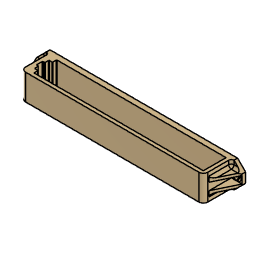
Porta Fusivel single v1 (Autodesk Fusion 360 design; units mm, degrees)
Autodesk Fusion 360 part; units mm, degrees
sketch "Sketch1" plane through (0, 0, 0) normal (0, 0, 1) x (1, 0, 0)
  line L0 (0, 0) -> (197, 0)
  line L1 (197, 0) -> (197, 25.5)
  line L2 (197, 25.5) -> (0, 25.5)
  line L3 (0, 25.5) -> (0, 0)
  line L4 (6.5, 25.5) -> (6.5, 20.8)
  line L5 (6.5, 20.8) -> (2.5, 20.8)
  line L6 (0, 12.75) -> (197, 12.75) construction
  line L7 (197, 17.5) -> (188, 17.5)
  line L8 (188, 17.5) -> (188, 8)
  line L9 (188, 8) -> (197, 8)
  line L10 (6.5, 4.7) -> (2.5, 4.7)
  line L11 (6.5, 0) -> (6.5, 4.7)
  line L12 (2.5, 20.8) -> (2.5, 16.25)
  line L13 (2.5, 16.25) -> (0, 16.25)
  line L14 (2.5, 4.7) -> (2.5, 9.25)
  line L15 (2.5, 9.25) -> (0, 9.25)
  line L16 (0, 25.5) -> (0, 51)
  line L17 (0, 51) -> (197, 51)
  line L18 (6.5, 46.3) -> (2.5, 46.3)
  line L19 (6.5, 51) -> (6.5, 46.3)
  line L20 (2.5, 41.75) -> (0, 41.75)
  line L21 (2.5, 46.3) -> (2.5, 41.75)
  line L22 (6.5, 25.5) -> (6.5, 30.2)
  line L23 (6.5, 30.2) -> (2.5, 30.2)
  line L24 (2.5, 30.2) -> (2.5, 34.75)
  line L25 (2.5, 34.75) -> (0, 34.75)
  line L26 (197, 33.5) -> (188, 33.5)
  line L27 (188, 33.5) -> (188, 43)
  line L28 (188, 43) -> (197, 43)
  line L29 (197, 51) -> (197, 25.5)
  line L30 (201, -4) -> (201, 25.5)
  line L31 (201, 55) -> (201, 25.5)
  line L32 (-4, 55) -> (201, 55)
  line L33 (-4, 25.5) -> (-4, 55)
  line L34 (-4, 25.5) -> (-4, -4)
  line L35 (-4, -4) -> (201, -4)
  line L36 (201, 21.5) -> (-4, 21.5)
  point P0 (0, 25.5)
  dimension "d1" = 25.5
  dimension "d2" = 197
  dimension "d5" = 4.7
  dimension "d6" = 4
  dimension "d7" = 9
  dimension "d8" = 9.5
  dimension "d9" = 2.5
  dimension "d10" = 7
  dimension "d19" = 4
  dimension "d74" = 4
  constraint horizontal L0
  constraint vertical L1
  constraint horizontal L2
  constraint vertical L3
  constraint coincident L0.start L3.end
  constraint coincident P0 L2
  constraint coincident P0 L3
  constraint coincident L3.end L0
  constraint coincident L0.start L3
  constraint coincident L2 L4.start
  constraint perpendicular L2 L4
  constraint perpendicular L3 L5
  constraint midpoint L3 L6.start
  constraint perpendicular L3 L6
  constraint midpoint L1 L6.end
  constraint coincident L1 L7.start
  constraint perpendicular L1 L7
  constraint perpendicular L6 L8
  constraint coincident L1 L9.end
  constraint perpendicular L1 L9
  constraint symmetric L6 L7 L9
  constraint symmetric L4.start L6 L11.start
  constraint symmetric L4.end L6 L10.start
  constraint symmetric L5.end L6 L10.end
  constraint perpendicular L5 L12
  constraint coincident L3 L13.end
  constraint perpendicular L3 L13
  constraint symmetric L6 L12.end L14.end
  constraint symmetric L6 L13.end L15.end
  constraint coincident P0 L2.end
  constraint coincident L0.end L1.start
  constraint symmetric L2 P0 L3.start
  constraint symmetric L2 L1.end L29.end
  constraint symmetric L2 L0.end L17.end
  constraint symmetric L2 L0.start L16.end
  constraint symmetric L2 L4.start L22.start
  constraint symmetric L2 L4.end L22.end
  constraint symmetric L2 L5.end L23.end
  constraint symmetric L2 L7.start L26.start
  constraint symmetric L2 L7.end L26.end
  constraint symmetric L2 L8.end L27.end
  constraint symmetric L2 L9.end L28.end
  constraint symmetric L2 L10.start L18.start
  constraint symmetric L2 L10.end L18.end
  constraint symmetric L2 L11.start L19.start
  constraint symmetric L2 L12.end L24.end
  constraint symmetric L2 L13.end L25.end
  constraint symmetric L2 L14.end L20.start
  constraint symmetric L2 L15.end L20.end
  constraint coincident L31 L36.start
  constraint coincident L33 L36.end
  constraint perpendicular L33 L36
  measures "d1" distance of L0.start P0
  measures "d2" distance of L1 L3
  measures "d5" distance of L4.start L4.end
  measures "d6" distance of L4.end L5.end
  measures "d7" distance of L7.start L7.end
  measures "d8" distance of L7.end L8.end
  measures "d9" distance of L12.end L13.end
  measures "d10" distance of L13 L15
  measures "d74" distance of L2 L36
extrude "Extrude1" add sketch "Sketch1" against normal blind 2 contours L1 L3 L16 L17 L29 L30 L31 L32 L33 L34 L36 | L2 L3 L4 L36 | L2 L16 L22 L23 L24 L25 | L1 L2 L4 L36 | L16 L17 L18 L19 L20 L21 | L26 L27 L28 L29
extrude "Extrude2" add sketch "Sketch1" along normal blind 9 contours L26 L27 L28 L29
extrude "Extrude3" add sketch "Sketch1" along normal blind 27 contours L1 L3 L16 L17 L29 L30 L31 L32 L33 L34 L36 | L2 L3 L4 L36 | L2 L16 L22 L23 L24 L25 | L1 L2 L4 L36 | L16 L17 L18 L19 L20 L21
fillet "Fillet1" radius 0.5 16 edges at (2.5, 34.75, 12.5) (2.5, 30.2, 12.5) (6.5, 46.3, 12.5) (2.5, 46.3, 12.5) (2.5, 41.75, 12.5) (6.5, 51, 12.5) (0, 41.75, 12.5) (0, 34.75, 12.5) (188, 43, 3.5) (188, 33.5, 3.5) (197, 51, 12.5) (197, 25.5, 12.5) (197, 43, 3.5) (197, 33.5, 3.5) (6.5, 25.5, 12.5) (6.5, 30.2, 12.5)
fillet "Fillet3" radius 5 2 edges at (201, 21.5, 12.5) (-4, 21.5, 12.5)
sketch "Sketch3" plane through (0, 0, -2) normal (0, 0, -1) x (1, 0, 0)
  line L0 (-4, -26.5) -> (-4, -55)
  line L1 (-4, -55) -> (201, -55)
  line L2 (201, -55) -> (201, -26.5)
  line L3 (197, -43.5) -> (197, -50.5)
  line L4 (196.5, -33.5) -> (188.5, -33.5)
  arc A0 (188.5, -33.5) -> (188, -34) centre (188.5, -34) ccw
  line L5 (188, -34) -> (188, -42.5)
  arc A1 (188, -42.5) -> (188.5, -43) centre (188.5, -42.5) ccw
  line L6 (188.5, -43) -> (196.5, -43)
  line L7 (196.5, -51) -> (7, -51)
  arc A2 (6.5, -50.5) -> (7, -51) centre (7, -50.5) ccw
  line L8 (6.5, -50.5) -> (6.5, -46.8)
  arc A3 (6.5, -46.8) -> (6, -46.3) centre (6, -46.8) ccw
  line L9 (6, -46.3) -> (3, -46.3)
  arc A4 (2.5, -45.8) -> (3, -46.3) centre (3, -45.8) ccw
  line L10 (2.5, -45.8) -> (2.5, -42.25)
  arc A5 (2.5, -42.25) -> (2, -41.75) centre (2, -42.25) ccw
  line L11 (2, -41.75) -> (0.5, -41.75)
  arc A6 (0, -41.25) -> (0.5, -41.75) centre (0.5, -41.25) ccw
  line L12 (0, -41.25) -> (0, -35.25)
  arc A7 (0.5, -34.75) -> (0, -35.25) centre (0.5, -35.25) ccw
  line L13 (0.5, -34.75) -> (2, -34.75)
  arc A8 (2, -34.75) -> (2.5, -34.25) centre (2, -34.25) ccw
  line L14 (2.5, -34.25) -> (2.5, -30.7)
  arc A9 (3, -30.2) -> (2.5, -30.7) centre (3, -30.7) ccw
  line L15 (3, -30.2) -> (6, -30.2)
  line L16 (6.5, -29.7) -> (6.5, -26)
  line L17 (7, -25.5) -> (196.5, -25.5)
  line L18 (196, -21.5) -> (1, -21.5)
  arc A10 (196.5, -51) -> (197, -50.5) centre (196.5, -50.5) ccw
  arc A11 (197, -26) -> (196.5, -25.5) centre (196.5, -26) ccw
  line L19 (197, -26) -> (197, -33)
  arc A12 (1, -21.5) -> (-4, -26.5) centre (1, -26.5) ccw
  arc A13 (201, -26.5) -> (196, -21.5) centre (196, -26.5) ccw
  arc A14 (6, -30.2) -> (6.5, -29.7) centre (6, -29.7) ccw
  arc A15 (7, -25.5) -> (6.5, -26) centre (7, -26) ccw
  arc A16 (196.5, -33.5) -> (197, -33) centre (196.5, -33) ccw
  arc A17 (197, -43.5) -> (196.5, -43) centre (196.5, -43.5) ccw
  line L20 (188.5, -44.65) -> (195.35, -44.65)
  line L21 (195.35, -44.65) -> (195.35, -49.35)
  line L22 (195.35, -49.35) -> (8.15, -49.35)
  line L23 (8.15, -49.35) -> (8.15, -46.8)
  arc A18 (8.15, -46.8) -> (6, -44.65) centre (6, -46.8) ccw
  line L24 (6, -44.65) -> (4.15, -44.65)
  line L25 (4.15, -44.65) -> (4.15, -42.25)
  arc A19 (4.15, -42.25) -> (2, -40.1) centre (2, -42.25) ccw
  line L26 (2, -40.1) -> (1.65, -40.1)
  line L27 (1.65, -40.1) -> (1.65, -36.4)
  line L28 (1.65, -36.4) -> (2, -36.4)
  arc A20 (2, -36.4) -> (4.15, -34.25) centre (2, -34.25) ccw
  line L29 (4.15, -34.25) -> (4.15, -31.85)
  line L30 (4.15, -31.85) -> (6, -31.85)
  arc A21 (6, -31.85) -> (8.15, -29.7) centre (6, -29.7) ccw
  line L31 (8.15, -29.7) -> (8.15, -27.15)
  line L32 (8.15, -27.15) -> (195.35, -27.15)
  line L33 (195.35, -27.15) -> (195.35, -31.85)
  line L34 (195.35, -31.85) -> (188.5, -31.85)
  arc A22 (188.5, -31.85) -> (186.35, -34) centre (188.5, -34) ccw
  line L35 (186.35, -34) -> (186.35, -42.5)
  arc A23 (186.35, -42.5) -> (188.5, -44.65) centre (188.5, -42.5) ccw
  dimension "d24" = 2
  dimension "d77" = 1.65
extrude "Extrude4" add sketch "Sketch3" against normal blind 2 contours L3 L4 A0 L5 A1 L6 L7 A2 L8 A3 L9 A4 L10 A5 L11 A6 L12 A7 L13 A8 L14 A9 L15 L16 L17 A10 A11 L19 A14 A15 A16 A17
sketch "Sketch4" plane through (0, 0, 27) normal (0, 0, 1) x (-1, 0, 0)
  arc A0 (-2, -41.75) -> (-2.5, -42.25) centre (-2, -42.25) ccw
  line L0 (-2.5, -42.25) -> (-2.5, -45.8)
  arc A1 (-3, -46.3) -> (-2.5, -45.8) centre (-3, -45.8) ccw
  line L1 (-3, -46.3) -> (-6, -46.3)
  arc A2 (-6, -46.3) -> (-6.5, -46.8) centre (-6, -46.8) ccw
  line L2 (-6.5, -46.8) -> (-6.5, -50.5)
  arc A3 (-7, -51) -> (-6.5, -50.5) centre (-7, -50.5) ccw
  line L3 (-7, -51) -> (-196.5, -51)
  line L4 (-197, -50.5) -> (-197, -26)
  line L5 (-6.5, -26) -> (-6.5, -29.7)
  line L6 (-6, -30.2) -> (-3, -30.2)
  arc A4 (-2.5, -30.7) -> (-3, -30.2) centre (-3, -30.7) ccw
  line L7 (-2.5, -30.7) -> (-2.5, -34.25)
  arc A5 (-2.5, -34.25) -> (-2, -34.75) centre (-2, -34.25) ccw
  line L8 (-2, -34.75) -> (-0.5, -34.75)
  arc A6 (0, -35.25) -> (-0.5, -34.75) centre (-0.5, -35.25) ccw
  line L9 (0, -35.25) -> (0, -41.25)
  arc A7 (-0.5, -41.75) -> (0, -41.25) centre (-0.5, -41.25) ccw
  line L10 (-0.5, -41.75) -> (-2, -41.75)
  line L11 (-201, -26.5) -> (-201, -55)
  line L12 (-201, -55) -> (4, -55)
  line L13 (4, -55) -> (4, -26.5)
  line L14 (-7, -51) -> (4, -51)
  line L15 (-196.5, -51) -> (-201, -51)
  line L16 (-1, -21.5) -> (-196, -21.5)
  line L17 (-196.5, -25.5) -> (-7, -25.5)
  arc A8 (-197, -50.5) -> (-196.5, -51) centre (-196.5, -50.5) ccw
  arc A9 (-196.5, -25.5) -> (-197, -26) centre (-196.5, -26) ccw
  arc A10 (4, -26.5) -> (-1, -21.5) centre (-1, -26.5) ccw
  arc A11 (-196, -21.5) -> (-201, -26.5) centre (-196, -26.5) ccw
  arc A12 (-6.5, -29.7) -> (-6, -30.2) centre (-6, -29.7) ccw
  arc A13 (-6.5, -26) -> (-7, -25.5) centre (-7, -26) ccw
  constraint coincident A3.start L3.start
  constraint coincident L13 L14.end
  constraint tangent A3 L14
  constraint coincident L3.end L15.start
  constraint coincident L11 L15.end
extrude "Extrude8" add 1 faces at (132.6667, 55, 17.3333) along direction (0, 1, 0) blind 2
sketch "Sketch6" plane through (0, 57, 0) normal (0, 1, 0) x (-1, 0, 0)
  line L0 (-201, 27) -> (-201, -2)
  line L1 (-201, -2) -> (4, -2)
  line L2 (4, -2) -> (4, 27)
  line L3 (4, 27) -> (-201, 27)
  line L4 (4, 27) -> (7, 27)
  line L5 (7, 27) -> (16, 18)
  line L6 (16, 18) -> (16, 14.25)
  line L7 (16, 14.25) -> (10, 14.25)
  arc A0 (10, 14.25) -> (10, 10.75) centre (10, 12.5) ccw
  line L8 (10, 12.5) -> (4, 12.5) construction
  line L9 (4, -2) -> (7, -2)
  line L10 (7, -2) -> (16, 7)
  line L11 (16, 7) -> (16, 10.75)
  line L12 (16, 10.75) -> (10, 10.75)
  line L13 (-98.5, 27) -> (-98.5, 53.5133) construction
  line L14 (-201, 27) -> (-204, 27)
  line L15 (-213, 18) -> (-213, 14.25)
  line L16 (-213, 14.25) -> (-207, 14.25)
  arc A1 (-207, 10.75) -> (-207, 14.25) centre (-207, 12.5) ccw
  line L17 (-204, 27) -> (-213, 18)
  line L18 (-201, -2) -> (-204, -2)
  line L19 (-204, -2) -> (-213, 7)
  line L20 (-213, 7) -> (-213, 10.75)
  line L21 (-213, 10.75) -> (-207, 10.75)
  line L22 (-213, 14.25) -> (-213, 10.75)
  arc A2 (-208, 14.25) -> (-208, 10.75) centre (-208, 12.5) ccw
  arc A3 (11, 10.75) -> (11, 14.25) centre (11, 12.5) ccw
  line L23 (16, 14.25) -> (16, 10.75)
  line L24 (16, 18) -> (4, 18)
  dimension "d41" = 6
  dimension "d43" = 3.5
  dimension "d44" = 3
  dimension "d45" = 135
  dimension "d46" = 12
  dimension "d50" = 1
  constraint coincident L2.end L3.start
  constraint perpendicular L2 L4
  constraint perpendicular L4 L6
  constraint perpendicular L6 L7
  constraint tangent L7 A0
  constraint coincident A0.centre L8.start
  constraint midpoint L2 L8.end
  constraint horizontal L8
  constraint symmetric L2.end L8 L1.end
  constraint symmetric L4.end L8 L9.end
  constraint symmetric L5.end L8 L10.end
  constraint symmetric L6.end L8 L11.end
  constraint symmetric L7.end L8 A0.end
  constraint coincident A0.end L12.end
  constraint midpoint L3 L13.start
  constraint perpendicular L3 L13
  constraint symmetric L2.end L13 L0.start
  constraint symmetric L4.end L13 L14.end
  constraint symmetric L5.end L13 L15.start
  constraint symmetric L6.end L13 L15.end
  constraint symmetric L7.end L13 L16.end
  constraint symmetric A0.end L13 A1.start
  constraint symmetric A0 L13 A1
  constraint symmetric L1.end L13 L0.end
  constraint symmetric L9.end L13 L18.end
  constraint symmetric L10.end L13 L19.end
  constraint symmetric L11.end L13 L20.end
  constraint tangent L21 A2
  constraint coincident L21 A2.end
  constraint coincident L16 A2.start
  constraint tangent L16 A2
  constraint symmetric L13 A2.start A3.end
  constraint symmetric L13 A2.end A3.start
  constraint symmetric L13 A2 A3
  constraint coincident L2 L24.end
  constraint perpendicular L2 L24
  measures "d41" distance of A0.centre L8.end
  measures "d43" distance of L7.end A0.end
  measures "d44" distance of L2.end L4.end
  measures "d45" angle of L5 L6
  measures "d46" distance of L2 L6
  measures "d50" distance of A1.centre A2.centre
extrude "Extrude9" add sketch "Sketch6" against normal blind 4 contours L0 L14 L15 L16 A1 L17 L18 L19 L20 L21 | L2 L4 L5 L24 | L2 L6 L7 A0 L9 L10 L11 L12 L24 | L16 L21 L22 A2 | L7 L12 A3 L23
chamfer "Chamfer2" distance 2.2 angle 45 8 edges at (-10.5, 53, 14.25) (-8.25, 53, 12.5) (-10.5, 53, 10.75) (-12.75, 53, 12.5) (209.75, 53, 12.5) (207.5, 53, 10.75) (205.25, 53, 12.5) (207.5, 53, 14.25)
sketch "Sketch8" plane through (0, 53, 0) normal (0, -1, 0) x (1, 0, 0)
  line L0 (-7, -2) -> (-4, -2)
  line L1 (-4, -2) -> (-4, 27)
  line L2 (-4, 27) -> (-7, 27)
  line L3 (-7, 27) -> (-16, 18)
  line L4 (-16, 18) -> (-16, 7)
  line L5 (-16, 7) -> (-7, -2)
  line L6 (-11, 16.45) -> (-10, 16.45)
  arc A0 (-10, 8.55) -> (-10, 16.45) centre (-10, 12.5) ccw
  line L7 (-10, 8.55) -> (-11, 8.55)
  arc A1 (-11, 16.45) -> (-11, 8.55) centre (-11, 12.5) ccw
  line L8 (-16, 16.65) -> (-4, 16.65)
  line L9 (-14.35, 19.65) -> (-4, 19.65)
  line L10 (-16, 8.35) -> (-4, 8.35)
  line L11 (-14.35, 5.35) -> (-4, 5.35)
  line L12 (-4, 27) -> (201, 27)
  line L13 (204, 27) -> (201, 27)
  line L14 (201, 27) -> (201, -2)
  line L15 (201, -2) -> (204, -2)
  line L16 (204, -2) -> (213, 7)
  line L17 (213, 7) -> (213, 18)
  line L18 (213, 18) -> (204, 27)
  arc A2 (208, 8.55) -> (208, 16.45) centre (208, 12.5) ccw
  line L19 (208, 8.55) -> (207, 8.55)
  arc A3 (207, 16.45) -> (207, 8.55) centre (207, 12.5) ccw
  line L20 (207, 16.45) -> (208, 16.45)
  line L21 (98.5, 27) -> (98.5, 42.1012) construction
  line L22 (211.35, 19.65) -> (201, 19.65)
  line L23 (213, 16.65) -> (201, 16.65)
  line L24 (213, 8.35) -> (201, 8.35)
  line L25 (211.35, 5.35) -> (201, 5.35)
  point P0 (201, 27)
  dimension "d60" = 3
  dimension "d61" = 0.2
  dimension "d71" = 3
  constraint coincident L4 L8.start
  constraint coincident L1 L8.end
  constraint perpendicular L1 L8
  constraint coincident L3 L9.start
  constraint coincident L1 L9.end
  constraint perpendicular L1 L9
  constraint coincident L4 L10.start
  constraint coincident L1 L10.end
  constraint perpendicular L1 L10
  constraint coincident L1 L11.end
  constraint perpendicular L1 L11
  constraint coincident L5 L11.start
  constraint equal L9 L11
  constraint coincident L1.end L2.start
  constraint midpoint L12 L21.start
  constraint perpendicular L12 L21
  constraint symmetric L8.start L21 L23.start
  constraint symmetric L8.end L21 L23.end
  constraint symmetric L9.start L21 L22.start
  constraint symmetric L9.end L21 L22.end
  constraint symmetric L10.start L21 L24.start
  constraint symmetric L10.end L21 L24.end
  constraint symmetric L11.start L21 L25.start
  constraint symmetric L11.end L21 L25.end
  measures "d60" distance of L8 L9
  measures "d61" distance of L6 L8
  measures "d71" distance of L10 L11
extrude "Extrude12" add sketch "Sketch8" along normal blind 0.2 contours L1 L4 L5 L10 L11 | L1 L3 L4 L8 L9 | L14 L17 L18 L22 L23 | L14 L16 L17 L24 L25
chamfer "Chamfer3" distance 25 distance2 12 4 edges at (-4, 52.8, 18.15) (-4, 52.8, 6.85) (201, 52.8, 18.15) (201, 52.8, 6.85) measured on face at (-4, 35.2667, 13.8833) measured on face at (-4, 35.2667, 13.8833) measured on face at (201, 35.2667, 13.8833) measured on face at (201, 35.2667, 13.8833)
fillet "Fillet5" radius 3 12 edges at (-9.175, 53, 19.65) (-4, 40.4, 19.65) (-4, 53, 23.325) (-4, 53, 1.675) (-9.175, 53, 5.35) (-4, 40.4, 5.35) (206.175, 53, 19.65) (201, 53, 23.325) (201, 40.4, 19.65) (201, 40.4, 5.35) (206.175, 53, 5.35) (201, 53, 1.675)
ref_plane "WorkPlane3" through (98.5, 41.75, 12.5) normal (-1, 0, 0) x (0, 1, 0)
equation "d2 = 94.5 mm + 94.5 mm + 4 mm + 4 mm"
